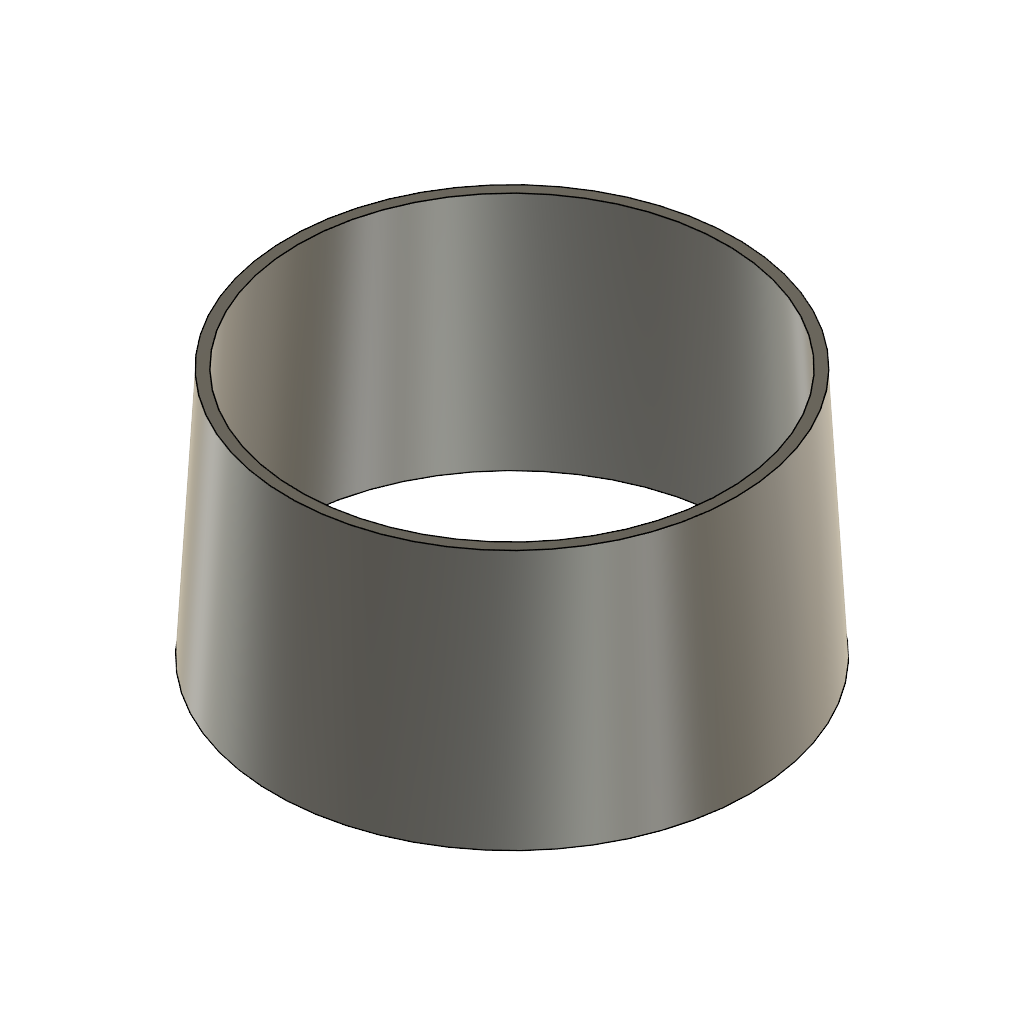
F360_Connector_model (Autodesk Fusion 360 design; units mm, degrees)
part number: 2026-09-23-12-14-58-906
Autodesk Fusion 360 part; units mm, degrees
sketch "Sketch1" plane through (0, 0, 0) normal (0, 0, 1) x (1, 0, 0)
  circle A0 centre (0, 0) radius 68.5
  dimension "d1" = 137
  constraint coincident A0.centre origin
  measures "d1" diameter of A0
ref_plane "WorkPlane1" through (0, 0, 72) normal (0, 0, 1) x (1, 0, 0)
sketch "Sketch2" plane through (0, 0, 72) normal (0, 0, 1) x (1, 0, 0)
  circle A0 centre (0, 0) radius 64.5
  dimension "d4" = 129
  constraint coincident A0.centre origin
  measures "d4" diameter of A0
loft "Loft1" add profiles "Sketch1", "Sketch2" section 1 section 2
shell "Shell1" thickness 3 removed faces 2 at (31.7275, 12.1488, 72) at (16.738, 15.5306, 0)
